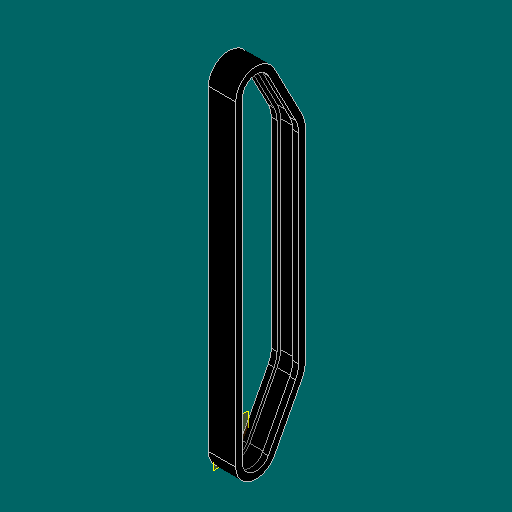
# Autodesk Inventor part: GĄ
Saved by Autodesk Inventor 2023 (Build 270158000, 158)
## iProperties
Created: 2023-01-28
Part Number: GĄ
Material: Generic
Document SubType Name: Modeling
Designer: HeavyDrewno
Density: 1 g/cm^3
Appearance: Anodized - Black
Author: HeavyDrewno
Autodesk Inventor part; units mm, degrees
ref_plane "YZ Plane" through (0, 0, 0) normal (1, 0, 0) x (0, 1, 0)
ref_plane "XZ Plane" through (0, 0, 0) normal (0, 1, 0) x (-1, 0, 0)
ref_plane "XY Plane" through (0, 0, 0) normal (0, 0, 1) x (1, 0, 0)
ref_plane "Work Plane1" through (-124.803, -23.6889, 361.6358) normal (-1, 0, 0) x (0, 0, 1)
sketch "Sketch1" plane through (-124.803, -23.6889, 361.6358) normal (-1, 0, 0) x (0, 0, 1)
  circle A0 centre (-46.5, 188.3919) radius 87.5 construction
  circle A1 centre (-46.5, 383.3919) radius 87.5 construction
  circle A2 centre (-46.5, 578.3919) radius 87.5 construction
  circle A3 centre (-46.5, 773.3919) radius 87.5 construction
  circle A4 centre (0, 943.8919) radius 50 construction
  circle A5 centre (0, 18.8919) radius 7 construction
  arc A6 (-44.2859, -4.3193) -> (50, 18.8919) centre (0, 18.8919) ccw
  arc A7 (50, 943.8919) -> (-44.3482, 966.9839) centre (0, 943.8919) ccw
  line L0 (50, 943.8919) -> (50, 18.8919)
  line L1 (-124.0003, 147.7724) -> (-44.2859, -4.3193)
  arc A8 (-134, 188.3919) -> (-124.0003, 147.7724) centre (-46.5, 188.3919) ccw
  arc A9 (-124.1093, 813.803) -> (-134, 773.3919) centre (-46.5, 773.3919) ccw
  line L2 (-44.3482, 966.9839) -> (-124.1093, 813.803)
  line L3 (-134, 773.3919) -> (-134, 188.3919)
  point P0 (-361.6358, 23.6889)
  dimension "d0" = 100
  constraints: 8 end point, 8 point on circle, 7 tangent, 4 centre point, 4 coincident, 2 concentric, 2 vertical, 4 other
  measures "d0" diameter of A6
ref_plane "Work Plane2" through (-124.803, -4.797, 361.6358) normal (0, 1, 0) x (-1, 0, 0)
sketch "Sketch2" plane through (-124.803, -4.797, 361.6358) normal (0, 1, 0) x (-1, 0, 0)
  line L0 (-62.0075, -25) -> (-62.0075, 25) construction
  line L1 (-7.2075, -25) -> (-7.2075, 25) construction
  line L2 (-14.615, 41) -> (-14.615, -134) construction
  line L3 (-54.615, 41) -> (-54.615, -134) construction
  line L4 (-14.615, 41) -> (-54.615, 41) construction
  line L5 (-69.215, -25) -> (-69.215, 25) construction
  line L6 (0, 50) -> (-69.215, 50) construction
  line L7 (-74.115, 50) -> (5.885, 50) construction
  line L8 (-94.115, 19.5) -> (-94.115, 95.5) construction
  line L9 (-74.115, 50) -> (-74.115, 40)
  line L10 (-74.115, 40) -> (-57.115, 40)
  line L11 (-57.115, 40) -> (-57.115, 50)
  line L12 (5.885, 50) -> (5.885, 40)
  line L13 (5.885, 40) -> (-11.115, 40)
  line L14 (-11.115, 40) -> (-11.115, 50)
  line L15 (-57.115, 50) -> (-11.115, 50)
  line L16 (5.885, 50) -> (5.885, 60)
  line L17 (5.885, 60) -> (-74.115, 60)
  line L18 (-74.115, 60) -> (-74.115, 50)
  point P0 (-124.803, -361.6358)
  point P1 (0, 50)
  dimension "d1" = 80
  dimension "d2" = 20
  dimension "d3" = 0
  dimension "d4" = 10
  dimension "d5" = 17
  dimension "d6" = 10
  dimension "d7" = 17
  dimension "d8" = 10
  constraints: 26 end point, 6 perpendicular, 3 horizontal, 3 point on line, 2 vertical, 1 collinear, 1 parallel
  measures "d1" distance of L7.start L7.end
  measures "d2" distance from line of L8 L7.start
  measures "d3" distance between parallel lines of L6 L7
  measures "d4" distance of L7.start L9.end
  measures "d5" distance of L9.end L10.end
  measures "d6" distance of L7.end L12.end
  measures "d7" distance of L12.end L13.end
  measures "d8" distance of L7.end L16.end
sweep "Sweep1" add profiles "Sketch2" path "Sketch1"
body "Solid1"
